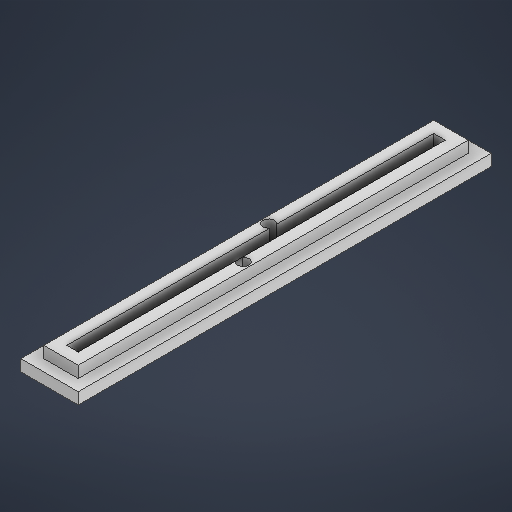
# Autodesk Inventor part: single_cell_top_case
Saved by Autodesk Inventor 2026 (Build 300175050, 175E)
## iProperties
Created: 2025-06-13
Part Number: single_cell_top_case
Material: Generic
Document SubType Name: Modeling
Designer: hamth
Density: 1 g/cm^3
Appearance: Default
Author: hamth
Autodesk Inventor part; units mm, degrees
ref_plane "YZ Plane" through (0, 0, 0) normal (1, 0, 0) x (0, 1, 0)
ref_plane "XZ Plane" through (0, 0, 0) normal (0, 1, 0) x (-1, 0, 0)
ref_plane "XY Plane" through (0, 0, 0) normal (0, 0, 1) x (1, 0, 0)
sketch "Sketch1" plane through (0, 0, 0) normal (0, 1, 0) x (-1, 0, 0)
  line L0 (0, 0) -> (0, -114.3)
  line L1 (0, -114.3) -> (-15.875, -114.3)
  line L2 (-15.875, -114.3) -> (-15.875, 0)
  line L3 (-15.875, 0) -> (0, 0)
  dimension "d0" = 114.3
  dimension "d1" = 15.875
  constraints: 8 end point, 2 parallel, 1 perpendicular, 1 vertical
  measures "d0" distance of L1.end L2.end
  measures "d1" distance of L0.end L1.end
extrude "Extrusion1" add sketch "Sketch1" along normal blind 3.175
sketch "Sketch2" plane through (0, 3.175, 0) normal (0, 1, 0) x (1, 0, 0)
  line L0 (0, 0) -> (3.175, 0)
  line L1 (0, 0) -> (15.875, 0) projected
  line L2 (3.175, 0) -> (3.175, 3.175)
  line L3 (3.175, 3.175) -> (6.35, 3.175)
  line L4 (6.35, 3.175) -> (6.35, 111.125)
  line L5 (6.35, 111.125) -> (3.175, 111.125)
  line L6 (3.175, 111.125) -> (3.175, 3.175)
  line L7 (15.875, 0) -> (15.875, 114.3) projected
  dimension "d4" = 3.175
  dimension "d5" = 3.175
  dimension "d6" = 3.175
  dimension "d7" = 107.95
  constraints: 12 end point, 3 perpendicular, 2 parallel, 1 point on line
  measures "d4" distance of L0.start L0.end
  measures "d5" distance of L0.end L2.end
  measures "d6" distance of L4.end L5.end
  measures "d7" distance of L3.end L4.end
extrude "Extrusion2" add sketch "Sketch2" along normal blind 3.175
sketch "Sketch3" plane through (0, 3.175, 0) normal (0, 1, 0) x (1, 0, 0)
  line L0 (15.875, 0) -> (15.875, 114.3) projected
  line L1 (15.875, 0) -> (12.7, 0)
  line L2 (0, 0) -> (15.875, 0) projected
  line L3 (12.7, 0) -> (12.7, 3.175)
  line L4 (12.7, 3.175) -> (9.525, 3.175)
  line L5 (9.525, 3.175) -> (9.525, 111.125)
  line L6 (9.525, 111.125) -> (12.7, 111.125)
  line L7 (12.7, 111.125) -> (12.7, 3.175)
  dimension "d10" = 3.175
  dimension "d11" = 3.175
  dimension "d12" = 3.175
  dimension "d13" = 107.95
  constraints: 12 end point, 2 parallel, 2 perpendicular, 1 horizontal, 1 point on line
  measures "d10" distance of L0.start L1.end
  measures "d11" distance of L1.end L3.end
  measures "d12" distance of L5.end L6.end
  measures "d13" distance of L4.end L5.end
extrude "Extrusion3" add sketch "Sketch3" along normal blind 3.175
sketch "Sketch4" plane through (0, 3.175, 0) normal (0, 1, 0) x (1, 0, 0)
  line L0 (6.35, 3.175) -> (3.175, 3.175) projected
  line L1 (6.35, 3.175) -> (9.525, 3.175)
  line L2 (9.525, 3.175) -> (9.525, 6.35)
  line L3 (9.525, 6.35) -> (6.35, 6.35)
  line L4 (6.35, 6.35) -> (6.35, 3.175)
  point P0 (0, 0)
  dimension "d16" = 3.175
  dimension "d17" = 3.175
  constraints: 8 end point, 2 parallel, 1 horizontal, 1 perpendicular
  measures "d16" distance of L1.end L2.end
  measures "d17" distance of L2.end L3.end
extrude "Extrusion4" add sketch "Sketch4" along normal blind 3.175
sketch "Sketch5" plane through (0, 3.175, 0) normal (0, 1, 0) x (1, 0, 0)
  line L0 (6.35, 6.35) -> (6.35, 111.125) projected
  line L1 (6.35, 111.125) -> (9.525, 111.125)
  line L2 (9.525, 111.125) -> (9.525, 107.95)
  line L3 (9.525, 107.95) -> (6.35, 107.95)
  line L4 (6.35, 107.95) -> (6.35, 111.125)
  point P0 (0, 0)
  dimension "d20" = 3.175
  dimension "d21" = 3.175
  constraints: 8 end point, 2 parallel, 1 horizontal, 1 perpendicular
  measures "d20" distance of L1.end L2.end
  measures "d21" distance of L2.end L3.end
extrude "Extrusion5" add sketch "Sketch5" along normal blind 3.175
sketch "Sketch6" plane through (0, 3.175, 0) normal (0, 1, 0) x (1, 0, 0)
  line L0 (0, 0) -> (7.9375, 0)
  line L1 (0, 0) -> (15.875, 0) projected
  line L2 (7.9375, 0) -> (7.9375, 57.15)
  dimension "d24" = 7.9375
  dimension "d25" = 57.15
  constraints: 4 end point, 1 midpoint, 1 perpendicular
  measures "d24" distance of L0.start L0.end
  measures "d25" distance of L0.end L2.end
hole "Hole1" at (7.9375, 3.175, -57.15) direction (0, -1, 0) diameter 3.175 end through all
sketch "Sketch10" plane through (0, 0, 0) normal (0, -1, 0) x (1, 0, 0)
  line L0 (15.875, 0) -> (15.875, -114.3) projected
  line L1 (15.875, 0) -> (15.875, -50.8)
  line L2 (15.875, -50.8) -> (10.795, -50.8)
  point P0 (0, 0)
  dimension "d46" = 50.8
  dimension "d47" = 5.08
  constraints: 4 end point, 1 perpendicular, 1 point on line
  measures "d46" distance of L0.start L1.end
  measures "d47" distance of L1.end L2.end
hole "Hole3" at (10.795, 0, -50.8) direction (0, 1, 0) diameter 3.175 end through all
sketch "Sketch11" plane through (0, 0, 0) normal (0, -1, 0) x (1, 0, 0)
  line L0 (0, 0) -> (0, -63.5)
  line L1 (0, -114.3) -> (0, 0) projected
  line L2 (0, -63.5) -> (5.08, -63.5)
  dimension "d55" = 63.5
  dimension "d56" = 5.08
  constraints: 4 end point, 1 perpendicular, 1 point on line
  measures "d55" distance of L0.start L0.end
  measures "d56" distance of L0.end L2.end
hole "Hole4" at (5.08, 0, -63.5) direction (0, 1, 0) diameter 3.175 end through all
body "Solid1"
